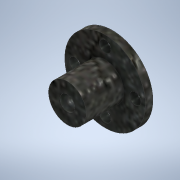
# Autodesk Inventor part: AcopleBrida4
Saved by Autodesk Inventor 2021 (Build 250183000, 183)
## iProperties
Created: 2022-10-28
Part Number: AcopleBrida4
Material: Acero
Document SubType Name: Modeling
Designer: zulet
Density: 7.85 g/cm^3
Appearance: Placa
Mass: 10.1847 g
Surface Area: 13.1249 cm^2
Volume: 1.29741 cm^3
Author: zulet
Autodesk Inventor part; units mm, degrees
ref_plane "YZ Plane" through (0, 0, 0) normal (1, 0, 0) x (0, 1, 0)
ref_plane "XZ Plane" through (0, 0, 0) normal (0, 1, 0) x (-1, 0, 0)
ref_plane "XY Plane" through (0, 0, 0) normal (0, 0, 1) x (1, 0, 0)
sketch "Sketch1" plane through (0, 0, 0) normal (0, 0, 1) x (1, 0, 0)
  circle A0 centre (0, 0) radius 10.7 projected
  circle A1 centre (8, 0) radius 1.5 projected
  circle A2 centre (0, 8) radius 1.5 projected
  circle A3 centre (0, -8) radius 1.5 projected
  circle A4 centre (0, 0) radius 2 projected
  circle A5 centre (-8, 0) radius 1.5 projected
extrude "Extrusion1" add sketch "Sketch1" along normal blind 2
sketch "Sketch2" plane through (0, 0, 2) normal (0, 0, 1) x (1, 0, 0)
  circle A0 centre (0, 0) radius 2 projected
  circle A1 centre (0, 0) radius 5
  dimension "d2" = 10
  constraints: 1 centre point, 1 coincident
  measures "d2" diameter of A1
extrude "Extrusion2" add sketch "Sketch2" along normal blind 10
body "Solid1"
